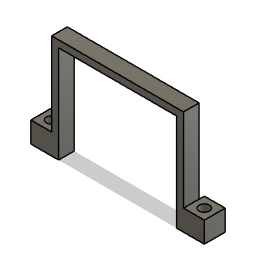
Fixation batterie (Autodesk Fusion 360 design; units mm, degrees)
Autodesk Fusion 360 part; units mm, degrees
sketch "Sketch1" plane through (0, 0, 0) normal (0, 0, 1) x (1, 0, 0)
  line L0 (0, 0) -> (6, 0)
  line L1 (6, 0) -> (6, 6)
  line L2 (6, 6) -> (0, 6)
  line L3 (0, 6) -> (0, 0)
  line L4 (6, 0) -> (8, 0)
  line L5 (8, 0) -> (8, 30)
  line L6 (8, 30) -> (6, 30)
  line L7 (6, 30) -> (6, 0)
  line L8 (6, 30) -> (25, 30)
  line L9 (25, 30) -> (25, 28)
  line L10 (25, 28) -> (6, 28)
  line L11 (6, 28) -> (6, 30)
  line L12 (50, 6) -> (50, 0)
  line L13 (44, 6) -> (50, 6)
  line L14 (44, 0) -> (42, 0)
  line L15 (50, 0) -> (44, 0)
  line L16 (44, 30) -> (25, 30)
  line L17 (42, 0) -> (42, 30)
  line L18 (44, 0) -> (44, 6)
  line L19 (44, 30) -> (44, 0)
  line L20 (25, 28) -> (44, 28)
  line L21 (44, 28) -> (44, 30)
  line L22 (42, 30) -> (44, 30)
  point P0 (50, 0)
  dimension "d1" = 6
  dimension "d2" = 6
  dimension "d3" = 2
  dimension "d4" = 30
  dimension "d5" = 19
  dimension "d6" = 2
  constraint horizontal L0
  constraint vertical L1
  constraint horizontal L2
  constraint vertical L3
  constraint coincident L0.start L3.end
  constraint horizontal L4
  constraint vertical L5
  constraint horizontal L6
  constraint vertical L7
  constraint horizontal L8
  constraint vertical L9
  constraint horizontal L10
  constraint vertical L11
  constraint symmetric L0.start L9 L12.end
  constraint symmetric L0.start L9 P0
  constraint symmetric L0.end L9 L14.start
  constraint symmetric L1.end L9 L13.start
  constraint symmetric L2.end L9 L12.start
  constraint symmetric L4.end L9 L14.end
  constraint symmetric L5.end L9 L17.end
  constraint symmetric L6.end L9 L16.start
  constraint symmetric L8.end L9 L16.end
  constraint symmetric L10.start L9 L20.start
  constraint symmetric L10.end L9 L20.end
  measures "d1" distance of L0.start L0.end
  measures "d2" distance of L0.start L2.end
  measures "d3" distance of L0.end L4.end
  measures "d4" distance of L0.end L6.end
  measures "d5" distance of L6.end L8.end
  measures "d6" distance of L6.end L10.end
extrude "Extrude1" add sketch "Sketch1" along normal blind 3 and the other way blind 3 contours L0 L1 L2 L3 L7 | L12 L13 L15 L18 L19 makes body 1 at (0, 2, 1) makes body 2 at (46, 2, 3)
extrude "Extrude2" add sketch "Sketch1" along normal blind 1.5 and the other way blind 1.5 contours L1 L4 L5 L7 L10 | L5 L6 L7 L8 L10 L11 | L5 L8 L9 L10 | L9 L16 L17 L20 | L14 L17 L18 L19 L20 | L16 L17 L19 L20 L21 L22 bodies 1 2
sketch "Sketch2" plane through (0, 6, 0) normal (0, 1, 0) x (-1, 0, 0)
  line L0 (0, -3) -> (0, 3)
  line L1 (0, 3) -> (-6, 3)
  line L2 (-6, 3) -> (-6, 1.5)
  line L3 (-6, 1.5) -> (-6, -1.5)
  line L4 (-6, -1.5) -> (-6, -3)
  line L5 (-6, -3) -> (0, -3)
  circle A0 centre (-3, 0) radius 1.5
  circle A1 centre (-47, 0) radius 1.5
  line L6 (-50, -3) -> (-50, 3)
  line L7 (-44, -3) -> (-50, -3)
  dimension "d15" = 3
  dimension "d16" = 3
  dimension "d17" = 3
  dimension "d18" = 3
  dimension "d19" = 3
  dimension "d20" = 3
  measures "d15" diameter of A1
  measures "d16" diameter of A0
  measures "d17" distance of L5 A0.centre
  measures "d18" distance of L0 A0.centre
  measures "d19" distance of A1.centre L6
  measures "d20" distance of A1.centre L7
extrude "Extrude3" cut sketch "Sketch2" against normal blind 18 contours A0 | A1 bodies 1
extrude "Extrude4" add 1 faces at (7.3333, 11.3333, 1.5) along direction (0, 0, 1) blind 1.5 on bodies 1 bodies 1
